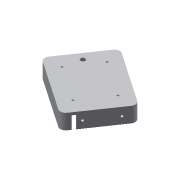
# Autodesk Inventor part: body2
Saved by Autodesk Inventor 2014 SP2 (Build 180246200, 246)
## iProperties
Created: 2016-01-20
Part Number: body2
Material: ABS plast
Document SubType Name: Modeling
Designer: Mervart
Mass: 35.1673 g
Surface Area: 339.189 cm^2
Volume: 33.1767 cm^3
Density: 1.06 g/cm^3
Appearance: Hliník – plochý
LastSaveDate: 21.09.2010
Hmotnost: 0
Author: Mervart
Autodesk Inventor part; units mm, degrees
ref_plane "YZ Plane" through (0, 0, 0) normal (1, 0, 0) x (0, 1, 0)
ref_plane "XZ Plane" through (0, 0, 0) normal (0, 1, 0) x (-1, 0, 0)
ref_plane "XY Plane" through (0, 0, 0) normal (0, 0, 1) x (1, 0, 0)
sketch "Náčrt4" plane through (0, 0, 0) normal (0, 0, 1) x (1, 0, 0)
  arc A0 (54.4803, -180.1301) -> (52.3875, -169.0116) centre (47.8747, -175.6173) ccw projected
  line L0 (-21.9257, -118.2421) -> (52.3875, -169.0116) projected
  line L1 (54.4803, -180.1301) -> (14.9928, -237.9293) projected
  arc A1 (3.8744, -240.022) -> (14.9928, -237.9293) centre (8.3872, -233.4164) ccw projected
  line L2 (3.8744, -240.022) -> (-70.4388, -189.2525) projected
  arc A2 (-72.5316, -178.134) -> (-70.4388, -189.2525) centre (-65.926, -182.6469) ccw projected
  line L3 (-72.5316, -178.134) -> (-33.0442, -120.3349) projected
  arc A3 (-21.9257, -118.2421) -> (-33.0442, -120.3349) centre (-26.4385, -124.8477) ccw projected
  point P0 (0, 0)
extrude "Vysunutí1" add sketch "Náčrt4" against normal blind 2
sketch "Náčrt5" plane through (0, 0, -2) normal (0, 0, -1) x (-1, 0, 0)
  arc A0 (-52.3875, -169.0116) -> (-54.4803, -180.1301) centre (-47.8747, -175.6173) ccw projected
  line L0 (-54.4803, -180.1301) -> (-14.9928, -237.9293) projected
  arc A1 (-14.9928, -237.9293) -> (-3.8744, -240.022) centre (-8.3872, -233.4164) ccw projected
  line L1 (-3.8744, -240.022) -> (70.4388, -189.2525) projected
  arc A2 (70.4388, -189.2525) -> (72.5316, -178.134) centre (65.926, -182.6469) ccw projected
  line L2 (72.5316, -178.134) -> (33.0442, -120.3349) projected
  arc A3 (33.0442, -120.3349) -> (21.9257, -118.2421) centre (26.4385, -124.8477) ccw projected
  line L3 (21.9257, -118.2421) -> (-52.3875, -169.0116) projected
  line L4 (-13.3414, -236.8011) -> (-52.8289, -179.0019)
  arc A4 (-51.2593, -170.663) -> (-52.8289, -179.0019) centre (-47.8747, -175.6173) ccw
  line L5 (-51.2593, -170.663) -> (23.0539, -119.8935)
  arc A5 (31.3928, -121.4631) -> (23.0539, -119.8935) centre (26.4385, -124.8477) ccw
  line L6 (31.3928, -121.4631) -> (70.8802, -179.2622)
  arc A6 (69.3106, -187.6011) -> (70.8802, -179.2622) centre (65.926, -182.6469) ccw
  line L7 (69.3106, -187.6011) -> (-5.0026, -238.3706)
  arc A7 (-13.3414, -236.8011) -> (-5.0026, -238.3706) centre (-8.3872, -233.4164) ccw
  point P0 (0, 0)
  dimension "d2" = 2
  constraints: 8 end point, 8 point on circle, 4 centre point, 7 other
  measures "d2" distance between parallel lines of L0 L4
extrude "Vysunutí2" add sketch "Náčrt5" along normal blind 21
sketch "Náčrt7" plane through (14.9928, -237.9293, 0) normal (0.8257023, -0.5641062, 0) x (0.5641062, 0.8257023, 0)
  line L0 (70, 0) -> (0, 0) construction
  line L1 (0, 0) -> (0, -23) construction
  line L2 (70, -23) -> (0, -23) construction
  line L3 (70, 0) -> (70, -23) construction
  line L4 (5, -23) -> (10, -23)
  line L5 (10, -23) -> (10, -4)
  line L6 (10, -4) -> (5, -4)
  line L7 (5, -4) -> (5, -23)
  point P0 (188.0012, 0)
  dimension "d5" = 5
  dimension "d6" = 5
  dimension "d7" = 4
  constraints: 8 end point, 2 parallel, 1 horizontal, 1 perpendicular, 1 point on line
  measures "d5" distance of L5.end L6.end
  measures "d6" distance between parallel lines of L1 L7
  measures "d7" distance between parallel lines of L0 L6
extrude "Vysunutí3" cut sketch "Náčrt7" against normal blind 7
sketch "Náčrt8" plane through (-72.5316, -178.134, 0) normal (-0.8257023, 0.5641062, 0) x (0.5641062, 0.8257023, 0)
  line L0 (0, 0) -> (70, 0) construction
  line L1 (70, 0) -> (70, 23) construction
  line L2 (0, 23) -> (70, 23) construction
  line L3 (0, 0) -> (0, 23) construction
  line L4 (2.36, 23) -> (12.639, 23)
  line L5 (12.639, 23) -> (12.639, 4)
  line L6 (12.639, 4) -> (2.36, 4)
  line L7 (2.36, 4) -> (2.36, 23)
  point P0 (188.0012, 0)
  dimension "d10" = 2.36
  dimension "d11" = 10.279
  dimension "d12" = 4
  constraints: 8 end point, 2 parallel, 1 horizontal, 1 perpendicular, 1 point on line
  measures "d10" distance between parallel lines of L3 L7
  measures "d11" distance of L5.end L6.end
  measures "d12" distance between parallel lines of L0 L6
extrude "Vysunutí4" cut sketch "Náčrt8" against normal blind 17.75
sketch "Náčrt9" plane through (0, 0, -2) normal (0, 0, -1) x (-1, 0, 0)
  arc A0 (-51.2593, -170.663) -> (-52.8289, -179.0019) centre (-47.8747, -175.6173) ccw construction
  line L0 (-52.8289, -179.0019) -> (-13.3414, -236.8011) construction
  arc A1 (-13.3414, -236.8011) -> (-5.0026, -238.3706) centre (-8.3872, -233.4164) ccw construction
  line L1 (-5.0026, -238.3706) -> (69.3106, -187.6011) construction
  arc A2 (69.3106, -187.6011) -> (70.8802, -179.2622) centre (65.926, -182.6469) ccw construction
  line L2 (70.8802, -179.2622) -> (31.3928, -121.4631) construction
  arc A3 (31.3928, -121.4631) -> (23.0539, -119.8935) centre (26.4385, -124.8477) ccw construction
  line L3 (23.0539, -119.8935) -> (-51.2593, -170.663) construction
  line L4 (26.4385, -124.8477) -> (-8.3872, -233.4164) construction
  line L5 (65.926, -182.6469) -> (-47.8747, -175.6173) construction
  point P0 (0, 0)
  point P1 (21.8542, -139.1392)
  point P2 (50.9458, -181.7215)
  point P3 (-3.8029, -219.1249)
  point P4 (-32.8944, -176.5426)
  point P5 (9.0257, -179.1321)
  dimension "d15" = 42
  dimension "d16" = 42
  dimension "d17" = 42
  dimension "d18" = 42
  constraints: 4 end point, 4 point on line, 1 midpoint
  measures "d15" distance of point (21.854, -139.139) point (9.026, -179.132)
  measures "d16" distance of point (9.026, -179.132) point (50.946, -181.722)
  measures "d17" distance of point (9.026, -179.132) point (-32.894, -176.543)
  measures "d18" distance of point (-3.803, -219.125) point (9.026, -179.132)
hole "Díra1" [suppressed]
sketch "Náčrt10" plane through (0, 0, -2) normal (0, 0, -1) x (-1, 0, 0)
  arc A0 (-51.2593, -170.663) -> (-52.8289, -179.0019) centre (-47.8747, -175.6173) ccw construction
  line L0 (-52.8289, -179.0019) -> (-13.3414, -236.8011) construction
  arc A1 (-13.3414, -236.8011) -> (-5.0026, -238.3706) centre (-8.3872, -233.4164) ccw construction
  line L1 (-5.0026, -238.3706) -> (69.3106, -187.6011) construction
  arc A2 (69.3106, -187.6011) -> (70.8802, -179.2622) centre (65.926, -182.6469) ccw construction
  line L2 (70.8802, -179.2622) -> (31.3928, -121.4631) construction
  arc A3 (31.3928, -121.4631) -> (23.0539, -119.8935) centre (26.4385, -124.8477) ccw construction
  line L3 (23.0539, -119.8935) -> (-51.2593, -170.663) construction
  line L4 (26.4385, -124.8477) -> (-8.3872, -233.4164) construction
  line L5 (-8.3872, -233.4164) -> (65.926, -182.6469) construction
  line L6 (65.926, -182.6469) -> (-47.8747, -175.6173) construction
  line L7 (21.2434, -141.0436) -> (-39.8185, -182.7601) construction
  line L8 (21.2434, -141.0436) -> (52.2251, -186.3928) construction
  circle A4 centre (21.2434, -141.0436) radius 4
  point P0 (0, 0)
  point P1 (9.0257, -179.1321)
  point P2 (48.9496, -181.5982)
  point P3 (-30.8982, -176.6659)
  dimension "d26" = 40
  dimension "d27" = 49.1153
  dimension "d28" = 63.1482
  dimension "d29" = 8
  constraints: 10 end point, 5 point on line, 2 parallel, 1 centre point, 1 coincident, 1 midpoint, 1 perpendicular
  measures "d26" distance of point (9.026, -179.132) L7.start
  measures "d27" distance of point (48.95, -181.598) L7.start
  measures "d28" distance of point (-30.898, -176.666) L7.start
  measures "d29" diameter of A4
extrude "Vysunutí5" add sketch "Náčrt10" along normal blind 1
sketch "Náčrt11" plane through (-21.2434, -141.0436, -3) normal (0, 0, -1) x (-1, 0, 0)
  point P0 (-21.2434, 141.0436)
  point P1 (0, 0)
hole "Díra2" at (-21.2434, -141.0436, -3) direction (0, 0, 1) diameter 3 depth 3 countersink diameter 6 countersink angle 80
pattern_linear "Obdélníkové pole1" count 2 spacing 49.1152 along (-0.5641062, -0.8257023, 0) count 2 spacing 63.1482 along (0.8257023, -0.5641062, 0) of "Díra2", "Vysunutí5"
sketch "Náčrt12" plane through (13.3414, -236.8011, -2) normal (-0.8257023, 0.5641062, 0) x (0.5641062, 0.8257023, 0)
  line L0 (5, 2) -> (5, 21) construction
  line L1 (0, 21) -> (5, 21) construction
  line L2 (0, 0) -> (0, 21) construction
  line L3 (70, 0) -> (0, 0) construction
  line L4 (70, 0) -> (70, 21) construction
  line L5 (10, 21) -> (70, 21) construction
  line L6 (10, 21) -> (10, 2) construction
  line L7 (10, 2) -> (5, 2) construction
  line L8 (68.2923, 10.5) -> (12.9396, 10.5) construction
  circle A0 centre (60, 10.5) radius 5
  line L9 (57.2308, 8.9458) -> (57.2694, 12.1211)
  line L10 (57.2694, 12.1211) -> (60.0386, 13.6753)
  line L11 (60.0386, 13.6753) -> (62.7692, 12.0542)
  line L12 (62.7692, 12.0542) -> (62.7306, 8.8789)
  line L13 (62.7306, 8.8789) -> (59.9614, 7.3247)
  line L14 (59.9614, 7.3247) -> (57.2308, 8.9458)
  point P0 (188.0012, -2)
  point P1 (50, 10.5)
  dimension "d45" = 21
  dimension "d46" = 10.5
  dimension "d47" = 70
  dimension "d48" = 10
  dimension "d49" = 10
  dimension "d50" = 10
  dimension "d51" = 3.1755
  dimension "d66" = 10.5
  constraints: 14 end point, 2 coincident, 2 point on line, 1 centre point, 1 parallel, 13 other
  measures "d45" distance between parallel lines of L5 L3
  measures "d46" distance between parallel lines of L8 L3
  measures "d47" distance between parallel lines of L2 L4
  measures "d48" distance from line of point (60, 10.5) L4
  measures "d49" distance of point (60, 10.5) point (50, 10.5)
  measures "d50" diameter of A0
  measures "d51" distance of L9.start point (60, 10.5)
  measures "d66" distance between parallel lines of L5 L8
extrude "Vysunutí6" add sketch "Náčrt12" along normal blind 2
sketch "Náčrt13" plane through (45.6475, -189.5135, -14.1211) normal (-0.8257023, 0.5641062, 0) x (0.4919221, 0.7200439, -0.4894379)
  line L0 (0, 0) -> (3.1755, 0) construction
  line L1 (3.1755, 0) -> (4.7632, -2.7501) construction
  line L2 (4.7632, -2.7501) -> (3.1755, -5.5001) construction
  line L3 (3.1755, -5.5001) -> (0, -5.5001) construction
  line L4 (0, -5.5001) -> (-1.5878, -2.7501) construction
  line L5 (-1.5878, -2.7501) -> (0, 0) construction
  circle A0 centre (1.5878, -2.7501) radius 5 construction
  circle A1 centre (1.5877, -2.7501) radius 1.55
  point P0 (107.0917, -76.2992)
  dimension "d54" = 3.1
  constraints: 1 centre point, 1 coincident
  measures "d54" diameter of A1
extrude "Vysunutí7" cut sketch "Náčrt13" against normal blind 8
pattern_linear "Obdélníkové pole2" count 2 spacing 43 along (-0.5641062, -0.8257023, 0) of "Vysunutí7", "Vysunutí6"
chamfer "Zkosení1" distance 2 angle 45 2 edges at (44.3673, -191.3874, -12.5) (20.1107, -226.8926, -12.5)
chamfer "Zkosení2" distance 1 angle 45 4 edges at (34.8982, -176.6659, -2) (7.192, -217.2205, -2) (-44.9496, -181.5982, -2) (-17.2434, -141.0436, -2)
sketch "Náčrt14" plane through (0, 0, -2) normal (0, 0, -1) x (-1, 0, 0)
  circle A0 centre (48.9496, -181.5982) radius 5 construction
  circle A1 centre (-30.8982, -176.6659) radius 5 construction
  arc A2 (-51.2593, -170.663) -> (-52.8289, -179.0019) centre (-47.8747, -175.6173) ccw construction
  line L0 (-52.8289, -179.0019) -> (-13.3414, -236.8011) construction
  arc A3 (-13.3414, -236.8011) -> (-5.0026, -238.3706) centre (-8.3872, -233.4164) ccw construction
  line L1 (-5.0026, -238.3706) -> (69.3106, -187.6011) construction
  arc A4 (69.3106, -187.6011) -> (70.8802, -179.2622) centre (65.926, -182.6469) ccw construction
  line L2 (70.8802, -179.2622) -> (31.3928, -121.4631) construction
  arc A5 (31.3928, -121.4631) -> (23.0539, -119.8935) centre (26.4385, -124.8477) ccw construction
  line L3 (23.0539, -119.8935) -> (-51.2593, -170.663) construction
  circle A6 centre (-3.192, -217.2205) radius 5 construction
  circle A7 centre (21.2434, -141.0436) radius 5 construction
  point P0 (0, 0)
  point P1 (42.8795, -156.0037)
  dimension "d67" = 10
  dimension "d68" = 82
  dimension "d69" = 41
  measures "d67" distance from line of point (42.879, -156.004) L2
  measures "d68" distance between parallel lines of L1 L3
  measures "d69" distance from line of L3 point (42.879, -156.004)
hole "Díra3" at (-42.8795, -156.0037, -2) direction (0, 0, 1) diameter 7 depth 2
equation "\"d16\" = d15"
equation "\"d17\" = d15"
equation "\"d18\" = d15"
equation "\"d41\" = d27"
equation "\"d44\" = d28"
equation "\"d46\" = 0.5 * d45"
equation "\"d49\" = d48"
equation "\"d69\" = 0.5 * d68"
